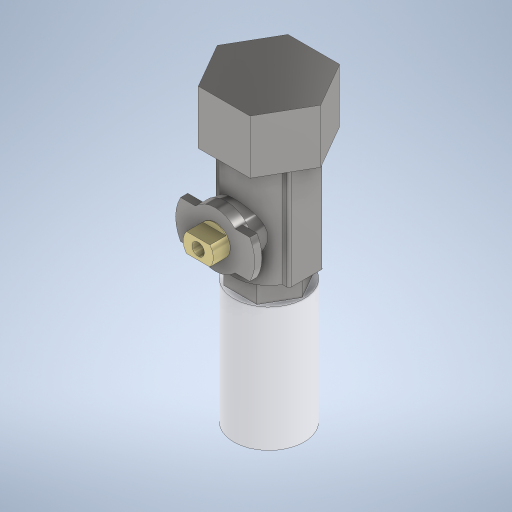
# Autodesk Inventor part: 가스벨브 역설계
Saved by Autodesk Inventor 2023.1 (Build 271208000, 208)
## iProperties
Created: 2022-08-14
Part Number: 가스벨브 역설계
Material: 일반
Document SubType Name: Modeling
Designer: fly01
Density: 1 g/cm^3
Appearance: 기본값
Author: fly01
Autodesk Inventor part; units mm, degrees
ref_plane "YZ Plane" through (0, 0, 0) normal (1, 0, 0) x (0, 1, 0)
ref_plane "XZ Plane" through (0, 0, 0) normal (0, 1, 0) x (-1, 0, 0)
ref_plane "XY Plane" through (0, 0, 0) normal (0, 0, 1) x (1, 0, 0)
sketch "스케치1" plane through (0, 0, 0) normal (0, 1, 0) x (-1, 0, 0)
  line L0 (12.5, 0) -> (6.25, -10.8253)
  line L1 (6.25, -10.8253) -> (-6.25, -10.8253)
  line L2 (-6.25, -10.8253) -> (-12.5, 0)
  line L3 (-12.5, 0) -> (-6.25, 10.8253)
  line L4 (-6.25, 10.8253) -> (6.25, 10.8253)
  line L5 (6.25, 10.8253) -> (12.5, 0)
  point P0 (0, 0)
  point P1 (0, 0)
  dimension "d0" = 25
  constraints: 12 end point, 1 coincident, 13 other
  measures "d0" distance of L2.end L0.start
extrude "돌출1" add sketch "스케치1" along normal blind 13
sketch "스케치2" plane through (0, 0, 0) normal (0, -1, 0) x (1, 0, 0)
  circle A0 centre (0, 0) radius 8.5
  line L0 (-9, 4.15) -> (9, 4.15)
  line L1 (9, 4.15) -> (9, -4.15)
  line L2 (9, -4.15) -> (-9, -4.15)
  line L3 (-9, -4.15) -> (-9, 4.15)
  line L4 (-9, 4.15) -> (9, -4.15) construction
  line L5 (9, 4.15) -> (-9, -4.15) construction
  point P0 (7.4181, -4.15)
  point P1 (7.4181, 4.15)
  point P2 (-7.4181, -4.15)
  point P3 (-7.4181, 4.15)
  dimension "d3" = 17
  dimension "d4" = 18
  dimension "d5" = 8.3
  constraints: 12 end point, 2 midpoint, 2 parallel, 1 centre point, 1 coincident, 1 horizontal, 1 perpendicular
  measures "d3" diameter of A0
  measures "d4" distance of L1.end L2.end
  measures "d5" distance of L0.end L1.end
extrude "돌출2" add sketch "스케치2" along normal blind 25
sketch "스케치3" plane through (0, -25, 0) normal (0, -1, 0) x (1, 0, 0)
  line L0 (8, 0) -> (4, -6.9282)
  line L1 (4, -6.9282) -> (-4, -6.9282)
  line L2 (-4, -6.9282) -> (-8, 0)
  line L3 (-8, 0) -> (-4, 6.9282)
  line L4 (-4, 6.9282) -> (4, 6.9282)
  line L5 (4, 6.9282) -> (8, 0)
  point P0 (0, 0)
  point P1 (0, 0)
  dimension "d8" = 16
  constraints: 12 end point, 1 coincident, 13 other
  measures "d8" distance of L0.start L2.end
extrude "돌출3" add sketch "스케치3" along normal blind 4.5
sketch "스케치4" plane through (0, -29.5, 0) normal (0, -1, 0) x (1, 0, 0)
  arc A0 (-7.4181, -4.15) -> (7.4181, -4.15) centre (0, 0) ccw projected
  circle A1 centre (0, 0) radius 8.5
  point P0 (7.4181, -4.15)
  dimension "d11" = 17
  constraints: 1 centre point, 1 coincident
  measures "d11" diameter of A1
extrude "돌출4" add sketch "스케치4" along normal blind 30
fillet "모깎기1" radius 0.5 4 edges at (-9, -12.5, 4.15) (9, -12.5, 4.15) (9, -12.5, -4.15) (-9, -12.5, -4.15)
sketch "스케치5" plane through (0, 0, 0) normal (1, 0, 0) x (0, 1, 0)
  line L0 (-8.2, 4) -> (-21.5, 4)
  line L1 (-21.5, 4) -> (-21.5, 13)
  line L2 (-21.5, 13) -> (-8.2, 13)
  line L3 (-8.2, 13) -> (-8.2, 4)
  line L4 (0, 8.5) -> (-25, 8.5) construction
  line L5 (-8.2, 4) -> (-21.5, 13) construction
  line L6 (-21.5, 4) -> (-8.2, 13) construction
  line L7 (-25, 8.5) -> (-25, 4.15) projected
  line L8 (-12.35, 13) -> (-17.35, 13)
  line L9 (-17.35, 13) -> (-17.35, 4)
  line L10 (-17.35, 4) -> (-12.35, 4)
  line L11 (-12.35, 4) -> (-12.35, 13)
  line L12 (-12.35, 13) -> (-17.35, 4) construction
  line L13 (-17.35, 13) -> (-12.35, 4) construction
  line L14 (-14.85, 13) -> (-14.85, 4)
  line L15 (-8.2, 4) -> (-14.5, 4)
  line L16 (-14.5, 4) -> (-14.5, 4.9729)
  line L17 (-14.5, 4.9729) -> (-8.2, 4.9729)
  line L18 (-8.2, 4.9729) -> (-8.2, 4)
  line L19 (-12.35, 4) -> (-12.35, 4.9729)
  line L20 (-14.5, 4.9729) -> (-17.35, 4.9729)
  line L21 (-17.35, 4.9729) -> (-17.35, 4)
  line L22 (-8.2, 13) -> (-8.2, 10.3)
  line L23 (-8.2, 10.3) -> (-9.2, 4.9729)
  point P0 (0, 0)
  point P1 (-14.85, 8.5)
  point P2 (-14.5, 7.2)
  point P3 (-14.85, 4.9729)
  point P4 (-12.35, 4.9729)
  dimension "d15" = 13.3
  dimension "d17" = 9
  dimension "d18" = 5
  dimension "d31" = 3.5
  dimension "d32" = 2.7
  dimension "d33" = 1
  constraints: 44 end point, 6 midpoint, 6 parallel, 5 perpendicular, 5 point on line, 4 horizontal
  measures "d15" distance of L1.end L2.end
  measures "d17" distance of L2.end L0.start
  measures "d18" distance between parallel lines of L11 L9
  measures "d31" distance between parallel lines of L7 L1
  measures "d32" distance of L2.end L22.end
  measures "d33" distance of L17.end L23.end
revolve "회전1" add sketch "스케치5" angle 360 about axis through (0, -14.85, 13) along (0, 0, -1) contours L0 L16 L17 L11 | L17 L20 L14 L2 L11 | L11 L2 L3 L23 L17
sketch "스케치8" plane through (0, -14.85, 13) normal (0, 0, 1) x (1, 0, 0)
  circle A0 centre (0, 0) radius 9.55
  line L0 (-9.55, 4.6) -> (9.55, 4.6)
  line L1 (9.55, 4.6) -> (9.55, -4.6)
  line L2 (9.55, -4.6) -> (-9.55, -4.6)
  line L3 (-9.55, -4.6) -> (-9.55, 4.6)
  line L4 (-9.55, 4.6) -> (9.55, -4.6) construction
  line L5 (9.55, 4.6) -> (-9.55, -4.6) construction
  circle A1 centre (0, 0) radius 6.65 projected
  point P0 (0, 14.85)
  point P1 (-4.8023, 4.6)
  point P2 (-8.3691, 4.6)
  point P3 (-8.3691, -4.6)
  point P4 (-4.8023, -4.6)
  point P5 (4.8023, -4.6)
  point P6 (8.3691, -4.6)
  point P7 (8.3691, 4.6)
  point P8 (4.8023, 4.6)
  dimension "d34" = 19.1
  dimension "d35" = 9.2
  constraints: 12 end point, 2 midpoint, 2 parallel, 1 centre point, 1 coincident, 1 horizontal, 1 perpendicular
  measures "d34" diameter of A0
  measures "d35" distance of L0.end L1.end
extrude "돌출7" add sketch "스케치8" against normal blind 1.75 contours A0 L2 A1 L0 | L0 A1 L2 A0 | A1 L2 L0 | L0 A1 | A1 L2
sketch "스케치9" plane through (-8.3691, -10.25, 13) normal (0, 0, 1) x (1, 0, 0)
  arc A0 (13.1715, 0) -> (3.5668, 0) centre (8.3691, -4.6) ccw projected
  circle A1 centre (8.3691, -4.6) radius 3.65
  line L0 (4.7191, -2.3) -> (12.0191, -2.3)
  line L1 (12.0191, -2.3) -> (12.0191, -6.9)
  line L2 (12.0191, -6.9) -> (4.7191, -6.9)
  line L3 (4.7191, -6.9) -> (4.7191, -2.3)
  line L4 (4.7191, -2.3) -> (12.0191, -6.9) construction
  line L5 (12.0191, -2.3) -> (4.7191, -6.9) construction
  point P0 (8.3691, 10.25)
  point P1 (5.535, -6.9)
  point P2 (11.2033, -6.9)
  point P3 (11.2033, -2.3)
  point P4 (5.535, -2.3)
  dimension "d38" = 7.3
  dimension "d39" = 4.6
  constraints: 12 end point, 2 midpoint, 2 parallel, 1 centre point, 1 coincident, 1 horizontal, 1 perpendicular
  measures "d38" diameter of A1
  measures "d39" distance of L0.end L1.end
extrude "돌출8" add sketch "스케치9" along normal blind 0.2 contours A1 L2 L0 | L0 A1 | A1 L2
extrude "돌출9" add sketch "스케치9" along normal blind 4.1 contours A1 L2 L0
sketch "스케치10" plane through (-8.3691, -10.25, 17.1) normal (0, 0, 1) x (1, 0, 0)
  arc A0 (11.2033, -6.9) -> (11.2033, -2.3) centre (8.3691, -4.6) ccw projected
  circle A1 centre (8.3691, -4.6) radius 1.5
  point P0 (8.3691, 10.25)
  dimension "d44" = 3
  constraints: 1 centre point, 1 coincident
  measures "d44" diameter of A1
extrude "돌출10" cut sketch "스케치10" against normal blind 4.1
sketch "스케치11" plane through (9, 0, 3.65) normal (1, 0, 0) x (0, 0, -1)
  point P0 (3.65, 0)
